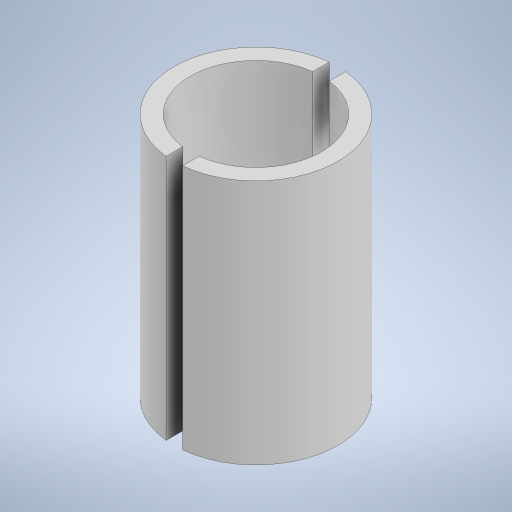
# Autodesk Inventor part: Forearm
Saved by Autodesk Inventor 2023 (Build 270158000, 158)
## iProperties
Created: 2023-03-21
Part Number: Forearm
Material: Generic
Document SubType Name: Modeling
Designer: 1senadi
Density: 1 g/cm^3
Appearance: Default
Author: 1senadi
Autodesk Inventor part; units mm, degrees
ref_plane "YZ Plane" through (0, 0, 0) normal (1, 0, 0) x (0, 1, 0)
ref_plane "XZ Plane" through (0, 0, 0) normal (0, 1, 0) x (-1, 0, 0)
ref_plane "XY Plane" through (0, 0, 0) normal (0, 0, 1) x (1, 0, 0)
sketch "Sketch1" plane through (0, 0, 0) normal (0, 1, 0) x (-1, 0, 0)
  circle A0 centre (0, 0) radius 50
  circle A1 centre (0, 0) radius 40
  line L0 (0, 50) -> (0, -50)
  line L1 (0, 0) -> (5, 0)
  line L2 (0, 0) -> (-5, 0)
  line L3 (5, 0) -> (5, -49.7494)
  line L4 (-5, 0) -> (-5, -49.7494)
  line L5 (5, 0) -> (5, 49.7494)
  line L6 (-5, 0) -> (-5, 49.7494)
  point P0 (-5, 39.6863)
  point P1 (-5, -39.6863)
  point P2 (5, 39.6863)
  point P3 (5, -39.6863)
  dimension "d0" = 100
  dimension "d1" = 80
  dimension "d2" = 5
  dimension "d3" = 5
  constraints: 14 end point, 6 point on circle, 3 vertical, 2 centre point, 2 coincident, 2 horizontal, 2 parallel
  measures "d0" diameter of A0
  measures "d1" diameter of A1
  measures "d2" distance of L1.start L1.end
  measures "d3" distance of L1.start L2.end
extrude "Extrusion1" add sketch "Sketch1" along normal blind 150 contours A0 L3 A1 L5 | L6 A1 L4 A0
body "Solid1"
